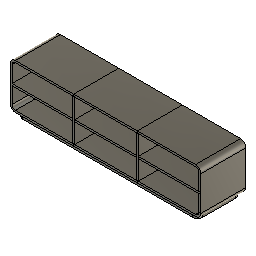
model-small (Autodesk Fusion 360 design; units mm, degrees)
Autodesk Fusion 360 part; units mm, degrees
sketch "Sketch1" plane through (0, 0, 0) normal (0, 1, 0) x (1, 0, 0)
  line L0 (0, 0) -> (1800, 0) construction
  line L1 (1800, 0) -> (1800, -425) construction
  line L2 (1800, -425) -> (0, -425) construction
  line L3 (0, -425) -> (0, 0) construction
  arc A0 (0, -375) -> (50, -425) centre (50, -375) ccw
  arc A1 (50, 0) -> (0, -50) centre (50, -50) ccw
  arc A2 (1800, -50) -> (1750, 0) centre (1750, -50) ccw
  arc A3 (1750, -425) -> (1800, -375) centre (1750, -375) ccw
  line L4 (600, -425) -> (600, 0) construction
  line L5 (1200, -425) -> (1200, 0) construction
  line L6 (0, -212.5) -> (600, -212.5) construction
  line L7 (600, -212.5) -> (1200, -212.5) construction
  line L8 (1800, -212.5) -> (1200, -212.5) construction
  line L9 (50, -425) -> (1750, -425)
  line L10 (1800, -375) -> (1800, -50)
  line L11 (1750, 0) -> (50, 0)
  line L12 (0, -50) -> (0, -375)
  arc A4 (1750, -407) -> (1782, -375) centre (1750, -375) ccw
  line L13 (1782, -375) -> (1782, -50)
  arc A5 (1782, -50) -> (1750, -18) centre (1750, -50) ccw
  line L14 (1750, -18) -> (50, -18)
  arc A6 (50, -18) -> (18, -50) centre (50, -50) ccw
  line L15 (18, -50) -> (18, -375)
  arc A7 (18, -375) -> (50, -407) centre (50, -375) ccw
  line L16 (50, -407) -> (1750, -407)
  line L17 (600, -407) -> (600, -425)
  line L18 (1200, -407) -> (1200, -425)
  line L19 (1200, -18) -> (1200, 0)
  line L20 (600, 0) -> (600, -18)
  line L21 (0, -212.5) -> (18, -212.5)
  line L22 (1782, -212.5) -> (1800, -212.5)
  line L23 (591, -407) -> (591, -18)
  line L24 (609, -407) -> (609, -18)
  line L25 (591, -407) -> (600, -212.5) construction
  line L26 (609, -407) -> (600, -212.5) construction
  line L27 (1191, -407) -> (1191, -18)
  line L28 (1209, -407) -> (1209, -18)
  line L29 (18, -221.5) -> (591, -221.5)
  line L30 (18, -203.5) -> (591, -203.5)
  line L31 (18, -221.5) -> (300, -212.5) construction
  line L32 (18, -203.5) -> (300, -212.5) construction
  line L33 (609, -221.5) -> (1191, -221.5)
  line L34 (609, -203.5) -> (1191, -203.5)
  line L35 (1209, -221.5) -> (1782, -221.5)
  line L36 (1209, -203.5) -> (1782, -203.5)
  line L37 (50, 0) -> (50, 40)
  line L38 (50, 40) -> (1750, 40)
  line L39 (1750, 40) -> (1750, 0)
  line L40 (900, 40) -> (900, 0) construction
  dimension "d4" = 425
  dimension "d5" = 1800
  dimension "d6" = 50
  dimension "d9" = 18
  dimension "d12" = 600
  dimension "d13" = 0
  dimension "d14" = 18
  dimension "d23" = 50
  dimension "d24" = 40
  constraint horizontal L0
  constraint vertical L1
  constraint horizontal L2
  constraint vertical L3
  constraint coincident L0.start L3.end
  constraint tangent L2 A0
  constraint coincident L2 A0.end
  constraint coincident L3 A0.start
  constraint tangent L0 A1
  constraint coincident L0 A1.start
  constraint coincident L3 A1.end
  constraint tangent L0 A2
  constraint coincident L1 A2.start
  constraint coincident L0 A2.end
  constraint tangent L2 A3
  constraint coincident L2 A3.start
  constraint coincident L1 A3.end
  constraint tangent L3 A0
  constraint tangent L3 A1
  constraint tangent L1 A2
  constraint tangent L1 A3
  constraint equal A0 A1
  constraint equal A1 A2
  constraint equal A2 A3
  constraint coincident L2 L4.start
  constraint coincident L0 L4.end
  constraint coincident L2 L5.start
  constraint coincident L0 L5.end
  constraint midpoint L3 L6.start
  constraint midpoint L4 L6.end
  constraint midpoint L5 L7.end
  constraint midpoint L1 L8.start
  constraint vertical L4
  constraint vertical L5
  constraint equal L6 L7
  constraint equal L7 L8
  constraint coincident L4 L17.start
  constraint coincident L16 L17.start
  constraint coincident L16 L18.start
  constraint coincident L5 L18.start
  constraint coincident L14 L19.start
  constraint coincident L5 L19.start
  constraint coincident L14 L20.end
  constraint coincident L4 L20.end
  constraint midpoint L15 L21.end
  constraint midpoint L13 L22.start
  constraint coincident L16 L23.start
  constraint coincident L14 L23.end
  constraint coincident L16 L24.start
  constraint coincident L14 L24.end
  constraint vertical L23
  constraint vertical L24
  constraint equal L25 L26
  constraint coincident L15 L29.start
  constraint coincident L23 L29.end
  constraint coincident L15 L30.start
  constraint coincident L23 L30.end
  constraint horizontal L29
  constraint horizontal L30
  constraint midpoint L6 L31.end
  constraint equal L31 L32
  constraint coincident L24 L33.start
  constraint coincident L27 L33.end
  constraint coincident L24 L34.start
  constraint coincident L27 L34.end
  constraint coincident L28 L35.start
  constraint coincident L13 L35.end
  constraint coincident L28 L36.start
  constraint coincident L13 L36.end
  constraint collinear L29 L33
  constraint collinear L33 L35
  constraint collinear L30 L34
  constraint collinear L34 L36
  constraint coincident L11 A2.end
  constraint vertical L37
  constraint horizontal L38
  constraint vertical L39
  constraint midpoint L38 L40.start
  constraint midpoint L0 L40.end
  constraint vertical L40
  measures "d4" distance of L0.start L2.end
  measures "d5" distance of L0.start L0.end
  measures "d6" radius of A0
  measures "d9" distance of L23 L24
  measures "d14" distance of L29.start L30.start
  measures "d23" horizontal distance of L0.start L37.end
  measures "d24" distance of A1.start L37.end
extrude "Extrude1" add sketch "Sketch1" along normal blind 425 contours A0 L9 L12 L15 A7 L16 L17 L21 | A3 L9 L10 A4 L13 L16 L18 L22 | L11 L14 L19 L20 | L24 L27 L33 L34 makes body 1 at (1000, 141.6667, 0) makes body 2 at (1383.3333, 141.6667, 407) makes body 3 at (233.3333, 141.6667, 407) makes body 4 at (803, 283.3333, 221.5)
extrude "Extrude2" add sketch "Sketch1" along normal blind 425 separate body contours A1 L11 L12 L14 A6 L15 L20 L21 | L9 L16 L17 L18 | A2 L10 L11 L13 A5 L14 L19 L22 makes body 5 at (416.6667, 141.6667, 0) makes body 6 at (800, 141.6667, 407) makes body 7 at (1566.6667, 141.6667, 0)
extrude "Extrude3" add sketch "Sketch1" along normal blind 425 contours L15 L23 L29 L30 | L13 L28 L35 L36 bodies 2 3 6 5 7
extrude "Extrude4" add sketch "Sketch1" along normal blind 425 separate body contours L14 L16 L23 L24 | L14 L16 L27 L28 makes body 8 at (1191, 283.3333, 277.3333) makes body 9 at (591, 283.3333, 277.3333)
extrude "Extrude5" add sketch "Sketch1" along normal up to surface (405 mm away) from surface at 20 separate body contours L11 L37 L38 L39 makes body 10
fillet "Fillet1" radius 50 4 edges at (50, 20, -20) (50, 425, -20) (1750, 20, -20) (1750, 425, -20) on bodies 10
sketch "Sketch3" plane through (0, 0, -40) normal (0, 0, -1) x (1, 0, 0)
  line L0 (100, -425) -> (1700, -425)
  line L1 (1750, -375) -> (1750, -70)
  line L2 (1700, -20) -> (100, -20)
  line L3 (50, -70) -> (50, -375)
  arc A0 (1700, -425) -> (1750, -375) centre (1700, -375) ccw
  arc A1 (1750, -70) -> (1700, -20) centre (1700, -70) ccw
  arc A2 (100, -20) -> (50, -70) centre (100, -70) ccw
  arc A3 (50, -375) -> (100, -425) centre (100, -375) ccw
  line L4 (100, -407) -> (1700, -407)
  arc A4 (1700, -407) -> (1732, -375) centre (1700, -375) ccw
  line L5 (1732, -375) -> (1732, -70)
  arc A5 (1732, -70) -> (1700, -38) centre (1700, -70) ccw
  line L6 (1700, -38) -> (100, -38)
  arc A6 (100, -38) -> (68, -70) centre (100, -70) ccw
  line L7 (68, -70) -> (68, -375)
  arc A7 (68, -375) -> (100, -407) centre (100, -375) ccw
extrude "Extrude6" cut sketch "Sketch3" against normal up to surface (40 mm away) contours L4 A4 L5 A5 L6 A6 L7 A7 bodies 10
equation "depth = 425 mm"
equation "unitWidth = 600 mm"
equation "bendRadius = 50 mm"
equation "d4 = depth"
equation "d5 = unitWidth * 3"
equation "d6 = bendRadius"
equation "d7 = -th"
equation "th = 18 mm"
equation "d9 = th"
equation "d12 = unitWidth"
equation "d14 = th"
equation "d15 = depth"
equation "d17 = depth"
equation "d19 = depth"
equation "d21 = depth"
equation "d23 = bendRadius"
equation "d33 = -th"
